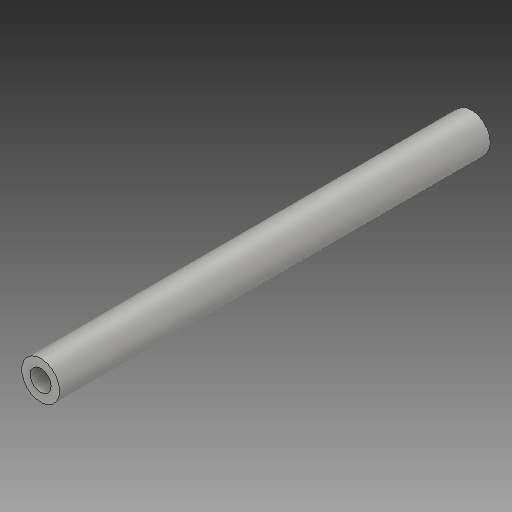
# Autodesk Inventor part: 342-03
Saved by Autodesk Inventor 2019 (Build 230136000, 136)
## iProperties
Company: Autodesk Inc.
Created: 2017-06-23
Part Number: 342-03
Material: Titanium
Document SubType Name: Modeling
Designer: Autodesk Inc.
Density: 4.51 g/cm^3
Appearance: Anodized - Light Gray
Mass: 48.3851 g
Surface Area: 81.0474 cm^2
Volume: 10.7284 cm^3
Author: Inventor
Autodesk Inventor part; units mm, degrees
ref_plane "YZ Plane" through (0, 0, 0) normal (1, 0, 0) x (0, 1, 0)
ref_plane "XZ Plane" through (0, 0, 0) normal (0, 1, 0) x (-1, 0, 0)
ref_plane "XY Plane" through (0, 0, 0) normal (0, 0, 1) x (1, 0, 0)
sketch "Sketch1" plane through (0, 0, 0) normal (0, 0, 1) x (1, 0, 0)
  circle A0 centre (0, 0) radius 6
  circle A1 centre (0, 0) radius 3.3
  dimension "d0" = 12
  dimension "d1" = 6.6
  constraints: 2 centre point, 2 coincident
  measures "d0" diameter of A0
  measures "d1" diameter of A1
extrude "Extrusion1" add sketch "Sketch1" along normal blind 136
body "Solid1"
